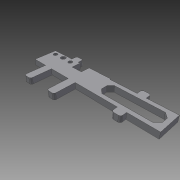
# Autodesk Inventor part: x_iddler_upper_nut_stop
Saved by Autodesk Inventor 2014 (Build 180170000, 170)
## iProperties
Created: 2013-12-02
Part Number: x_iddler_upper_nut_stop
Material: Generic
Document SubType Name: Modeling
Designer: buben
Density: 1 g/cm^3
Appearance: Default
Author: buben
Autodesk Inventor part; units mm, degrees
ref_plane "YZ Plane" through (0, 0, 0) normal (1, 0, 0) x (0, 1, 0)
ref_plane "XZ Plane" through (0, 0, 0) normal (0, 1, 0) x (-1, 0, 0)
ref_plane "XY Plane" through (0, 0, 0) normal (0, 0, 1) x (1, 0, 0)
sketch "Sketch1" plane through (0, 0, 0) normal (0, 0, 1) x (1, 0, 0)
  line L0 (0, 0) -> (128, 0)
  line L1 (128, 0) -> (128, 22)
  line L2 (0, 23) -> (0, 0)
  line L3 (68, 23) -> (68, 22)
  line L4 (68, 22) -> (128, 22)
  line L5 (33, 23) -> (33, 14)
  line L6 (33, 14) -> (44, 14)
  line L7 (44, 14) -> (44, 23)
  line L8 (68, 23) -> (44, 23)
  line L9 (33, 23) -> (0, 23)
  line L10 (72, 14) -> (72, 8)
  line L11 (72, 8) -> (76, 4)
  line L12 (76, 4) -> (120, 4)
  line L13 (120, 4) -> (124, 8)
  line L14 (124, 8) -> (124, 14)
  line L15 (124, 14) -> (120, 18)
  line L16 (120, 18) -> (76, 18)
  line L17 (76, 18) -> (72, 14)
  line L18 (68, 22) -> (68, 0) construction
  circle A0 centre (5.5, 18.5) radius 2.25
  circle A1 centre (25.5, 18.5) radius 2.25
  circle A2 centre (15.5, 19.099) radius 2.75
  circle A3 centre (38.5, 19.099) radius 7.5 construction
  circle A4 centre (38.5, 19.099) radius 4 construction
  point P0 (33, 18.5)
  dimension "d0" = 128
  dimension "d1" = 23
  dimension "d2" = 22
  dimension "d3" = 60
  dimension "d4" = 11
  dimension "d5" = 9
  dimension "d6" = 33
  dimension "d7" = 45
  dimension "d8" = 4
  dimension "d9" = 4
  dimension "d10" = 4
  dimension "d11" = 4
  dimension "d12" = 4
  dimension "d13" = 4.5
  dimension "d14" = 4.5
  dimension "d15" = 5.5
  dimension "d16" = 20
  dimension "d17" = 5.5
  dimension "d18" = 8
  dimension "d19" = 15
  dimension "d20" = 10
  constraints: 38 end point, 15 perpendicular, 6 parallel, 5 centre point, 3 horizontal alignment, 2 point on circle, 1 coincident, 1 collinear, 1 horizontal, 1 midpoint, 1 point on line
  measures "d0" distance of L0.start L0.end
  measures "d1" distance of L2.start L0.start
  measures "d2" distance of L0.end L1.end
  measures "d3" distance of L3.end L1.end
  measures "d4" distance of L5.end L6.end
  measures "d5" distance of L6.end L7.end
  measures "d6" distance of L5.start L2.start
  measures "d7" angle of L11 L10
  measures "d8" horizontal distance of L16.end L10.start
  measures "d9" distance between parallel lines of L18 L10
  measures "d10" distance between parallel lines of L1 L14
  measures "d11" distance between parallel lines of L4 L16
  measures "d12" distance between parallel lines of L0 L12
  measures "d13" diameter of A0
  measures "d14" diameter of A1
  measures "d15" distance from line of L2 A0.centre
  measures "d16" distance of A1.centre A0.centre
  measures "d17" diameter of A2
  measures "d18" diameter of A4
  measures "d19" diameter of A3
  measures "d20" horizontal distance of A0.centre A2.centre
extrude "Extrusion1" add sketch "Sketch1" along normal blind 6
sketch "Sketch2" plane through (0, 0, 6) normal (0, 0, 1) x (1, 0, 0)
  line L0 (0, 0) -> (128, 0) projected
  line L1 (128, 0) -> (128, 22) projected
  line L2 (128, 22) -> (68, 22) projected
  line L3 (33, 23) -> (0, 23) projected
  line L4 (0, 23) -> (0, 0) projected
  line L5 (22.5, 23) -> (30.5, 23)
  line L6 (30.5, 23) -> (30.5, 27)
  line L7 (28.5, 29) -> (24.5, 29)
  line L8 (22.5, 27) -> (22.5, 23)
  line L9 (94, 22) -> (102, 22)
  line L10 (102, 22) -> (102, 26)
  line L11 (100, 28) -> (96, 28)
  line L12 (94, 26) -> (94, 22)
  line L13 (15, 0) -> (23, 0)
  line L14 (23, 0) -> (23, -19)
  line L15 (21, -21) -> (17, -21)
  line L16 (15, -19) -> (15, 0)
  line L17 (44, 0) -> (52, 0)
  line L18 (52, 0) -> (52, -19)
  line L19 (50, -21) -> (46, -21)
  line L20 (44, -19) -> (44, 0)
  line L21 (94, 0) -> (102, 0)
  line L22 (102, 0) -> (102, -4)
  line L23 (100, -6) -> (96, -6)
  line L24 (94, -4) -> (94, 0)
  arc A0 (24.5, 29) -> (22.5, 27) centre (24.5, 27) ccw
  arc A1 (30.5, 27) -> (28.5, 29) centre (28.5, 27) ccw
  arc A2 (96, 28) -> (94, 26) centre (96, 26) ccw
  arc A3 (102, 26) -> (100, 28) centre (100, 26) ccw
  arc A4 (15, -19) -> (17, -21) centre (17, -19) ccw
  arc A5 (21, -21) -> (23, -19) centre (21, -19) ccw
  arc A6 (44, -19) -> (46, -21) centre (46, -19) ccw
  arc A7 (50, -21) -> (52, -19) centre (50, -19) ccw
  arc A8 (94, -4) -> (96, -6) centre (96, -4) ccw
  arc A9 (100, -6) -> (102, -4) centre (100, -4) ccw
  dimension "d23" = 2
  dimension "d24" = 8
  dimension "d25" = 8
  dimension "d26" = 8
  dimension "d27" = 8
  dimension "d28" = 8
  dimension "d29" = 21
  dimension "d30" = 6
  dimension "d31" = 6
  dimension "d32" = 22.5
  dimension "d33" = 26
  dimension "d34" = 15
  dimension "d35" = 21
  dimension "d38" = 6
  constraints: 40 end point, 20 point on circle, 20 tangent, 10 centre point, 10 parallel, 9 equal radius, 5 horizontal, 5 perpendicular, 5 point on line, 2 collinear
  measures "d23" radius of A0
  measures "d24" distance between parallel lines of L6 L8
  measures "d25" distance between parallel lines of L10 L12
  measures "d26" distance between parallel lines of L14 L16
  measures "d27" distance between parallel lines of L18 L20
  measures "d28" distance between parallel lines of L22 L24
  measures "d29" distance between parallel lines of L13 L15
  measures "d30" distance between parallel lines of L3 L7
  measures "d31" distance between parallel lines of L9 L11
  measures "d32" distance between parallel lines of L4 L8
  measures "d33" distance between parallel lines of L1 L10
  measures "d34" distance between parallel lines of L4 L16
  measures "d35" distance between parallel lines of L20 L14
  measures "d38" distance between parallel lines of L0 L23
extrude "Extrusion2" add sketch "Sketch2" against normal blind 6
body "Solid1"
